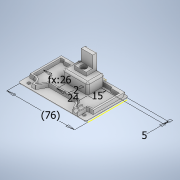
# Autodesk Inventor part: Deckel_Logo
Saved by Autodesk Inventor 2020 (Build 240168000, 168)
## iProperties
Created: 2020-09-26
Part Number: Deckel_Logo
Material: Generisch
Document SubType Name: Modeling
Designer: hpcwoess
Density: 1 g/cm^3
Appearance: Vorgabe
Author: hpcwoess
Autodesk Inventor part; units mm, degrees
ref_plane "YZ Plane" through (0, 0, 0) normal (1, 0, 0) x (0, 1, 0)
ref_plane "XY Plane" through (0, 0, 0) normal (0, 0, 1) x (1, 0, 0)
ref_plane "Arbeitsebene1" through (-34.5, -94, 30.7) normal (0, 1, 0) x (-1, 0, 0)
sketch "Skizze1" plane through (-34.5, -94, 30.7) normal (0, 1, 0) x (-1, 0, 0)
  circle A0 centre (-5, 5) radius 1.75 projected
  circle A1 centre (-67, 5) radius 1.75 projected
  arc A2 (-54.3246, 3.4866) -> (-54.0238, 3.1454) centre (-53.4437, 3.96) ccw projected
  line L0 (-54.3246, 3.4866) -> (-56.467, 7.4734) projected
  arc A3 (-56.467, 7.4734) -> (-57.3479, 8) centre (-57.3479, 7) ccw projected
  line L1 (-10, 8) -> (-14.6521, 8) projected
  arc A4 (-67, 0) -> (-65.2, 0.3352) centre (-67, 5) ccw projected
  line L2 (-67, 0) -> (-72, 0) projected
  line L3 (-72, 0) -> (-72, -34.5) projected
  line L4 (-62, -34.5) -> (-72, -34.5) projected
  line L5 (-62, -36) -> (-62, -34.5) projected
  line L6 (-62, -36) -> (-26, -36) projected
  line L7 (-26, -36) -> (-26, -34.5) projected
  line L8 (-9, -34.5) -> (-26, -34.5) projected
  line L9 (-9, -36) -> (-9, -34.5) projected
  line L10 (-9, -36) -> (-1, -36) projected
  arc A5 (-1, -36) -> (0, -35) centre (-1, -35) ccw projected
  line L11 (0, -35) -> (0, 0) projected
  line L12 (0, 0) -> (-5, 0) projected
  arc A6 (-10, 5) -> (-5, 0) centre (-5, 5) ccw projected
  line L13 (-10, 5) -> (-10, 8) projected
  arc A7 (-14.6521, 8) -> (-15.533, 7.4734) centre (-14.6521, 7) ccw projected
  line L14 (-15.533, 7.4734) -> (-20.4626, -1.7) projected
  line L15 (-24.2, -1.7) -> (-20.4626, -1.7) projected
  arc A8 (-24.2, -1.7) -> (-24.2487, -0.7) centre (-34.5, -1.7) ccw projected
  line L16 (-24.2487, -0.7) -> (-22.25, -0.7) projected
  line L17 (-22.25, 8) -> (-22.25, -0.7) projected
  line L18 (-22.25, 8) -> (-49.75, 8) projected
  line L19 (-49.75, -0.7) -> (-49.75, 8) projected
  line L20 (-49.75, -0.7) -> (-47, -0.7) projected
  line L21 (-47, -1.7) -> (-47, -0.7) projected
  line L22 (-50.4728, -1.7) -> (-47, -1.7) projected
  arc A9 (-50.4728, -1.7) -> (-54.0238, 3.1454) centre (-59.5709, -4.6437) ccw projected
  arc A10 (-74, -36) -> (-72, -38) centre (-72, -36) ccw projected
  line L23 (-74, -36) -> (-74, 8) projected
  arc A11 (-72, 10) -> (-74, 8) centre (-72, 8) ccw projected
  line L24 (-58.8, 10) -> (0, 10) projected
  arc A12 (2, 8) -> (0, 10) centre (0, 8) ccw projected
  line L25 (2, 8) -> (2, -36) projected
  arc A13 (0, -38) -> (2, -36) centre (0, -36) ccw projected
  line L26 (0, -38) -> (-72, -38) projected
  line L27 (-26.4, -35.6) -> (-61.6, -35.6)
  line L28 (-61.6, -35.6) -> (-61.6, -34.1)
  line L29 (-61.6, -34.1) -> (-71.6, -34.1)
  line L30 (-71.6, -34.1) -> (-71.6, -0.4)
  line L31 (-71.6, -0.4) -> (-67, -0.4)
  arc A14 (-67, -0.4) -> (-61.624, 4.4915) centre (-67, 5) ccw
  line L32 (-61.624, 4.4915) -> (-61.624, 7.6)
  line L33 (-61.624, 7.6) -> (-57.3479, 7.6)
  arc A15 (-56.8193, 7.284) -> (-57.3479, 7.6) centre (-57.3479, 7) ccw
  line L34 (-56.8193, 7.284) -> (-54.6769, 3.2973)
  arc A16 (-54.6769, 3.2973) -> (-54.2558, 2.8196) centre (-53.4437, 3.96) ccw
  arc A17 (-50.7686, -2.1) -> (-54.2558, 2.8196) centre (-59.5709, -4.6437) ccw
  line L35 (-50.7686, -2.1) -> (-46.6, -2.1)
  line L36 (-46.6, -2.1) -> (-46.6, -0.3)
  line L37 (-46.6, -0.3) -> (-49.35, -0.3)
  line L38 (-49.35, -0.3) -> (-49.35, 7.6)
  line L39 (-49.35, 7.6) -> (-22.65, 7.6)
  line L40 (-22.65, 7.6) -> (-22.65, -0.3)
  line L41 (-22.65, -0.3) -> (-24.6995, -0.3)
  arc A18 (-24.6081, -2.1) -> (-24.6995, -0.3) centre (-34.5, -1.7) ccw
  line L42 (-24.6081, -2.1) -> (-20.2235, -2.1)
  line L43 (-20.2235, -2.1) -> (-15.1807, 7.284)
  arc A19 (-14.6521, 7.6) -> (-15.1807, 7.284) centre (-14.6521, 7) ccw
  line L44 (-14.6521, 7.6) -> (-10.4, 7.6)
  line L45 (-10.4, 7.6) -> (-10.4, 5)
  arc A20 (-10.4, 5) -> (-5, -0.4) centre (-5, 5) ccw
  line L46 (-5, -0.4) -> (-0.4, -0.4)
  line L47 (-0.4, -0.4) -> (-0.4, -35)
  arc A21 (-1, -35.6) -> (-0.4, -35) centre (-1, -35) ccw
  line L48 (-1, -35.6) -> (-8.6, -35.6)
  line L49 (-8.6, -35.6) -> (-8.6, -34.1)
  line L50 (-8.6, -34.1) -> (-26.4, -34.1)
  line L51 (-26.4, -34.1) -> (-26.4, -35.6)
  line L52 (-59.6, -33.6) -> (-28.4, -33.6)
  line L53 (-28.4, -33.6) -> (-28.4, -32.1)
  line L54 (-28.4, -32.1) -> (-6.6, -32.1)
  line L55 (-6.6, -32.1) -> (-6.6, -33.6)
  line L56 (-6.6, -33.6) -> (-2.4, -33.6)
  line L57 (-2.4, -33.6) -> (-2.4, -2.4)
  line L58 (-2.4, -2.4) -> (-5, -2.4)
  arc A22 (-12.4, 5) -> (-5, -2.4) centre (-5, 5) ccw
  line L59 (-12.4, 5) -> (-12.4, 5.6)
  line L60 (-12.4, 5.6) -> (-13.8151, 5.6)
  line L61 (-13.8151, 5.6) -> (-19.0277, -4.1)
  line L62 (-19.0277, -4.1) -> (-26.9734, -4.1)
  arc A23 (-26.9734, -4.1) -> (-27.3691, 1.7) centre (-34.5, -1.7) ccw
  line L63 (-27.3691, 1.7) -> (-24.65, 1.7)
  line L64 (-24.65, 1.7) -> (-24.65, 5.6)
  line L65 (-24.65, 5.6) -> (-47.35, 5.6)
  line L66 (-47.35, 5.6) -> (-47.35, 1.7)
  line L67 (-47.35, 1.7) -> (-44.6, 1.7)
  line L68 (-44.6, 1.7) -> (-44.6, -4.1)
  line L69 (-44.6, -4.1) -> (-52.4291, -4.1)
  arc A24 (-52.4291, -4.1) -> (-55.416, 1.1905) centre (-59.5709, -4.6437) ccw
  arc A25 (-56.4387, 2.3505) -> (-55.416, 1.1905) centre (-53.4437, 3.96) ccw
  line L70 (-56.4387, 2.3505) -> (-58.1849, 5.6)
  line L71 (-58.1849, 5.6) -> (-59.624, 5.6)
  line L72 (-59.624, 5.6) -> (-59.624, 4.4046)
  arc A26 (-67, -2.4) -> (-59.624, 4.4046) centre (-67, 5) ccw
  line L73 (-67, -2.4) -> (-69.6, -2.4)
  line L74 (-69.6, -2.4) -> (-69.6, -32.1)
  line L75 (-69.6, -32.1) -> (-59.6, -32.1)
  line L76 (-59.6, -32.1) -> (-59.6, -33.6)
  line L77 (-65.2, 10) -> (-65.2, 0.3352) projected
  line L78 (-57.3479, 8) -> (-58.8, 8) projected
  line L79 (-58.8, 8) -> (-58.8, 10) projected
  line L80 (-72, 10) -> (-65.2, 10) projected
  line L81 (-58.8, 10) -> (-65.2, 10)
  line L82 (-58.8, 8) -> (-61.8, 8)
  line L83 (-61.8, 8) -> (-61.8, 4.5)
  point P0 (-34.5, -30.7)
  dimension "d0" = 0.4
  dimension "d1" = 2
  constraints: 106 end point, 26 point on circle, 13 centre point, 2 horizontal, 1 perpendicular, 57 other
  measures "d0" distance between parallel lines of L6 L27
  measures "d1" distance between parallel lines of L27 L52
extrude "Extrusion1" add sketch "Skizze1" against normal blind 2 contours L0 A3 L78 L79 L24 A12 L25 A13 L26 A10 L23 A11 L80 L77 A4 L2 L3 L4 L5 L6 L7 L8 L9 L10 A5 L11 L12 A6 L13 L1 A7 L14 L15 A8 L16 L17 L18 L19 L20 L21 L22 A9 A2 | A2 A9 L22 L21 L20 L19 L18 L17 L16 A8 L15 L14 A7 L1 L13 A6 L12 L11 A5 L10 L9 L8 L7 L6 L5 L4 L3 L2 A4 L77 L81 L79 L78 A3 L0 | L27 L28 L29 L30 L31 A14 L32 L33 A15 L34 A16 A17 L35 L36 L37 L38 L39 L40 L41 A18 L42 L43 A19 L44 L45 A20 L46 L47 A21 L48 L49 L50 L51 | L76 L75 L74 L73 A26 L72 L71 L70 A25 A24 L69 L68 L67 L66 L65 L64 L63 A23 L62 L61 L60 L59 A22 L58 L57 L56 L55 L54 L53 L52
sketch "Skizze4" plane through (-34.5, -94, 30.7) normal (0, 1, 0) x (-1, 0, 0)
  circle A0 centre (-5, 5) radius 1.75
  circle A1 centre (-67, 5) radius 1.75
  arc A2 (-54.3246, 3.4866) -> (-54.0238, 3.1454) centre (-53.4437, 3.96) ccw
  line L0 (-54.3246, 3.4866) -> (-56.467, 7.4734)
  arc A3 (-56.467, 7.4734) -> (-57.3479, 8) centre (-57.3479, 7) ccw
  line L1 (-57.3479, 8) -> (-62.024, 8)
  line L2 (-62.024, 8) -> (-62.024, 4.5108)
  arc A4 (-67, 0) -> (-62.024, 4.5108) centre (-67, 5) ccw
  line L3 (-67, 0) -> (-72, 0)
  line L4 (-72, 0) -> (-72, -34.5)
  line L5 (-62, -34.5) -> (-72, -34.5)
  line L6 (-62, -36) -> (-62, -34.5)
  line L7 (-62, -36) -> (-26, -36)
  line L8 (-26, -36) -> (-26, -34.5)
  line L9 (-9, -34.5) -> (-26, -34.5)
  line L10 (-9, -36) -> (-9, -34.5)
  line L11 (-9, -36) -> (-1, -36)
  arc A5 (-1, -36) -> (0, -35) centre (-1, -35) ccw
  line L12 (0, -35) -> (0, 0)
  line L13 (0, 0) -> (-5, 0)
  arc A6 (-10, 5) -> (-5, 0) centre (-5, 5) ccw
  line L14 (-10, 5) -> (-10, 8)
  line L15 (-10, 8) -> (-14.6521, 8)
  arc A7 (-14.6521, 8) -> (-15.533, 7.4734) centre (-14.6521, 7) ccw
  line L16 (-15.533, 7.4734) -> (-20.4626, -1.7)
  line L17 (-24.2, -1.7) -> (-20.4626, -1.7)
  arc A8 (-24.2, -1.7) -> (-24.2487, -0.7) centre (-34.5, -1.7) ccw
  line L18 (-24.2487, -0.7) -> (-22.25, -0.7)
  line L19 (-22.25, 8) -> (-22.25, -0.7)
  line L20 (-22.25, 8) -> (-49.75, 8)
  line L21 (-49.75, -0.7) -> (-49.75, 8)
  line L22 (-49.75, -0.7) -> (-47, -0.7)
  line L23 (-47, -1.7) -> (-47, -0.7)
  line L24 (-50.4728, -1.7) -> (-47, -1.7)
  arc A9 (-50.4728, -1.7) -> (-54.0238, 3.1454) centre (-59.5709, -4.6437) ccw
  arc A10 (-74, -36) -> (-72, -38) centre (-72, -36) ccw
  line L25 (-74, -36) -> (-74, 8)
  arc A11 (-72, 10) -> (-74, 8) centre (-72, 8) ccw
  line L26 (-72, 10) -> (0, 10)
  arc A12 (2, 8) -> (0, 10) centre (0, 8) ccw
  line L27 (2, 8) -> (2, -36)
  arc A13 (0, -38) -> (2, -36) centre (0, -36) ccw
  line L28 (0, -38) -> (-72, -38)
  line L29 (-26.4, -35.6) -> (-61.6, -35.6)
  line L30 (-61.6, -35.6) -> (-61.6, -34.1)
  line L31 (-61.6, -34.1) -> (-71.6, -34.1)
  line L32 (-71.6, -34.1) -> (-71.6, -0.4)
  line L33 (-71.6, -0.4) -> (-67, -0.4)
  arc A14 (-67, -0.4) -> (-61.624, 4.4915) centre (-67, 5) ccw
  line L34 (-61.624, 4.4915) -> (-61.624, 7.6)
  line L35 (-61.624, 7.6) -> (-57.3479, 7.6)
  arc A15 (-56.8193, 7.284) -> (-57.3479, 7.6) centre (-57.3479, 7) ccw
  line L36 (-56.8193, 7.284) -> (-54.6769, 3.2973)
  arc A16 (-54.6769, 3.2973) -> (-54.2558, 2.8196) centre (-53.4437, 3.96) ccw
  arc A17 (-50.7686, -2.1) -> (-54.2558, 2.8196) centre (-59.5709, -4.6437) ccw
  line L37 (-50.7686, -2.1) -> (-20.2235, -2.1)
  line L38 (-46.6, -0.3) -> (-49.35, -0.3)
  line L39 (-49.35, -0.3) -> (-49.35, 7.6)
  line L40 (-49.35, 7.6) -> (-22.65, 7.6)
  line L41 (-22.65, 7.6) -> (-22.65, -0.3)
  line L42 (-22.65, -0.3) -> (-24.6995, -0.3)
  line L43 (-24.6081, -2.1) -> (-20.2235, -2.1)
  line L44 (-20.2235, -2.1) -> (-15.1807, 7.284)
  arc A18 (-14.6521, 7.6) -> (-15.1807, 7.284) centre (-14.6521, 7) ccw
  line L45 (-14.6521, 7.6) -> (-10.4, 7.6)
  line L46 (-10.4, 7.6) -> (-10.4, 5)
  arc A19 (-10.4, 5) -> (-5, -0.4) centre (-5, 5) ccw
  line L47 (-5, -0.4) -> (-0.4, -0.4)
  line L48 (-0.4, -0.4) -> (-0.4, -35)
  arc A20 (-1, -35.6) -> (-0.4, -35) centre (-1, -35) ccw
  line L49 (-1, -35.6) -> (-8.6, -35.6)
  line L50 (-8.6, -35.6) -> (-8.6, -34.1)
  line L51 (-8.6, -34.1) -> (-26.4, -34.1)
  line L52 (-26.4, -34.1) -> (-26.4, -35.6)
  line L53 (-59.6, -33.6) -> (-28.4, -33.6)
  line L54 (-28.4, -33.6) -> (-28.4, -32.1)
  line L55 (-28.4, -32.1) -> (-6.6, -32.1)
  line L56 (-6.6, -32.1) -> (-6.6, -33.6)
  line L57 (-6.6, -33.6) -> (-2.4, -33.6)
  line L58 (-2.4, -33.6) -> (-2.4, -2.4)
  line L59 (-2.4, -2.4) -> (-5, -2.4)
  arc A21 (-12.4, 5) -> (-5, -2.4) centre (-5, 5) ccw
  line L60 (-12.4, 5) -> (-12.4, 5.6)
  line L61 (-12.4, 5.6) -> (-13.8151, 5.6)
  line L62 (-13.8151, 5.6) -> (-19.0277, -4.1)
  line L63 (-19.0277, -4.1) -> (-26.9734, -4.1)
  line L64 (-27.3691, 1.7) -> (-24.65, 1.7)
  line L65 (-24.65, 1.7) -> (-24.65, 5.6)
  line L66 (-24.65, 5.6) -> (-47.35, 5.6)
  line L67 (-47.35, 5.6) -> (-47.35, 1.7)
  line L68 (-47.35, 1.7) -> (-44.6, 1.7)
  line L69 (-19.0277, -4.1) -> (-52.4291, -4.1)
  arc A22 (-52.4291, -4.1) -> (-55.416, 1.1905) centre (-59.5709, -4.6437) ccw
  arc A23 (-56.4387, 2.3505) -> (-55.416, 1.1905) centre (-53.4437, 3.96) ccw
  line L70 (-56.4387, 2.3505) -> (-58.1849, 5.6)
  line L71 (-58.1849, 5.6) -> (-59.624, 5.6)
  line L72 (-59.624, 5.6) -> (-59.624, 4.4046)
  arc A24 (-67, -2.4) -> (-59.624, 4.4046) centre (-67, 5) ccw
  line L73 (-67, -2.4) -> (-69.6, -2.4)
  line L74 (-69.6, -2.4) -> (-69.6, -32.1)
  line L75 (-69.6, -32.1) -> (-59.6, -32.1)
  line L76 (-59.6, -32.1) -> (-59.6, -33.6)
  point P0 (-34.5, -30.7)
  point P1 (-34.5, -30.7)
  point P2 (-26.9734, -4.1)
  dimension "d4" = 0.4
  dimension "d5" = 2
  constraints: 154 end point, 46 point on circle, 25 centre point, 51 other
  measures "d4" distance between parallel lines of L7 L29
  measures "d5" distance between parallel lines of L29 L53
extrude "Extrusion2" add sketch "Skizze4" along normal blind 4 contours L29 L30 L31 L32 L33 A14 L34 L35 A15 L36 A16 A17 L37 L44 A18 L45 L46 A19 L47 L48 A20 L49 L50 L51 L52
sketch "Skizze5" plane through (-34.5, -96, 30.7) normal (0, -1, 0) x (1, 0, 0)
  line L0 (24, -18) -> (48, -18)
  line L1 (48, -18) -> (48, -33)
  line L2 (48, -33) -> (24, -33)
  line L3 (24, -33) -> (24, -18)
  line L4 (-2, 8) -> (-2, -36) projected
  line L5 (74, -36) -> (74, 8) projected
  line L6 (0, -38) -> (72, -38) projected
  line L7 (50, -16) -> (22, -16)
  line L8 (22, -16) -> (22, -35)
  line L9 (22, -35) -> (50, -35)
  line L10 (50, -35) -> (50, -16)
  point P0 (34.5, -30.7)
  dimension "d8" = 24
  dimension "d9" = 15
  dimension "d10" = 26
  dimension "d11" = 76
  dimension "d12" = 5
  dimension "d13" = 2
  constraints: 16 end point, 4 parallel, 2 perpendicular, 1 horizontal, 3 other
  measures "d8" distance of L0.start L0.end
  measures "d9" distance of L0.end L1.end
  measures "d10" distance between parallel lines of L4 L3
  measures "d11" distance between parallel lines of L5 L4
  measures "d12" distance between parallel lines of L2 L6
  measures "d13" distance between parallel lines of L0 L7
extrude "Extrusion3" add sketch "Skizze5" against normal blind 14 contours L0 L1 L2 L3 | L10 L9 L8 L7
extrude "Extrusion4" cut sketch "Skizze5" against normal blind 12 contours L0 L1 L2 L3
sketch "Skizze6" plane through (-34.5, -84, 30.7) normal (0, -1, 0) x (1, 0, 0)
  circle A0 centre (36, -25.5) radius 3.25
  line L0 (48, -18) -> (48, -33) projected
  line L1 (24, -18) -> (48, -18) projected
  line L2 (29.5, -21.75) -> (42.5, -21.75)
  line L3 (42.5, -21.75) -> (42.5, -29.25)
  line L4 (42.5, -29.25) -> (29.5, -29.25)
  line L5 (29.5, -29.25) -> (29.5, -21.75)
  line L6 (50, -35) -> (22, -35) projected
  line L7 (29.5, -29.25) -> (42.5, -29.25)
  line L8 (42.5, -29.25) -> (42.5, -35)
  line L9 (42.5, -35) -> (29.5, -35)
  line L10 (29.5, -35) -> (29.5, -29.25)
  point P0 (34.5, -30.7)
  dimension "d18" = 6.5
  dimension "d19" = 12
  dimension "d20" = 7.5
  dimension "d25" = 7.5
  dimension "d26" = 3.75
  dimension "d27" = 13
  dimension "d28" = 6.5
  constraints: 16 end point, 4 parallel, 2 horizontal, 2 perpendicular, 2 point on line, 1 centre point
  measures "d18" diameter of A0
  measures "d19" distance from line of A0.centre L0
  measures "d20" distance from line of L1 A0.centre
  measures "d25" distance between parallel lines of L2 L4
  measures "d26" distance from line of L4 A0.centre
  measures "d27" distance of L2.start L2.end
  measures "d28" distance from line of L3 A0.centre
sketch "Skizze7" plane through (37.1, -94, -3.4) normal (1, 0, 0) x (0, 0, -1)
  line L0 (1.5, 4) -> (0.9, 4) projected
  line L1 (3.9, 0) -> (3.9, -2) projected
  line L2 (1.5, 4) -> (3.9, 4)
  line L3 (3.9, 4) -> (3.9, 0)
  line L4 (3.9, 0) -> (1.5, 0)
  line L5 (1.5, 0) -> (1.5, 4)
  line L6 (3.9, 0) -> (2.2, 0)
  line L7 (2.2, 0) -> (2.2, 2.2)
  line L8 (2.2, 2.2) -> (3.9, 2.2)
  line L9 (3.9, 2.2) -> (3.9, 0)
  line L10 (0, 0) -> (0, 4) projected
  line L11 (1.5, 4) -> (0, 4)
  line L12 (0, 4) -> (0, 0)
  line L13 (0, 0) -> (1.5, 0)
  line L14 (1.5, 0) -> (1.5, 4)
  point P0 (-3.4, 94)
  point P1 (2.2, 0)
  point P2 (3.9, 2.2)
  point P3 (1.5, 0)
  dimension "d21" = 1.7
  dimension "d22" = 2.2
  constraints: 24 end point, 6 parallel, 3 horizontal, 3 perpendicular
  measures "d21" distance of L7.end L8.end
  measures "d22" distance of L6.end L7.end
extrude "Extrusion5" add sketch "Skizze7" against normal up to surface (71.2 mm away) contours L5 L13 L10 L11 L0 | L2 L3 L8 L7 L4 L5
sketch "Skizze8" plane through (-34.5, -96, 30.7) normal (0, -1, 0) x (1, 0, 0)
  point P0 (34.5, -30.7)
extrude "Extrusion6" add sketch "Skizze6" against normal blind 6 contours L2 L3 L4 L5
sketch "Skizze9" plane through (-34.5, -84, 30.7) normal (0, -1, 0) x (1, 0, 0)
  circle A0 centre (36, -25.5) radius 3.25
  line L0 (48, -18) -> (48, -33)
  line L1 (24, -18) -> (48, -18)
  line L2 (29.5, -21.75) -> (42.5, -21.75)
  line L3 (42.5, -21.75) -> (42.5, -29.25)
  line L4 (42.5, -29.25) -> (29.5, -29.25)
  line L5 (29.5, -29.25) -> (29.5, -21.75)
  line L6 (50, -35) -> (22, -35)
  line L7 (29.5, -29.25) -> (42.5, -29.25)
  line L8 (42.5, -29.25) -> (42.5, -35)
  line L9 (42.5, -35) -> (29.5, -35)
  line L10 (29.5, -35) -> (29.5, -29.25)
  point P0 (34.5, -30.7)
  point P1 (34.5, -30.7)
  dimension "d31" = 6.5
  dimension "d32" = 12
  dimension "d33" = 7.5
  dimension "d34" = 7.5
  dimension "d35" = 3.75
  dimension "d36" = 13
  dimension "d37" = 6.5
  constraints: 22 end point, 4 parallel, 2 horizontal, 2 perpendicular, 2 point on line, 1 centre point
  measures "d31" diameter of A0
  measures "d32" distance from line of A0.centre L0
  measures "d33" distance from line of L1 A0.centre
  measures "d34" distance between parallel lines of L2 L4
  measures "d35" distance from line of L4 A0.centre
  measures "d36" distance of L2.start L2.end
  measures "d37" distance from line of L3 A0.centre
extrude "Extrusion7" add sketch "Skizze9" against normal blind 19 contours L4 L8 L6 L10
sketch "Skizze10" plane through (-34.5, -78, 30.7) normal (0, 1, 0) x (1, 0, 0)
  line L0 (29.5, 21.75) -> (42.5, 21.75) projected
  line L1 (42.5, 21.75) -> (42.5, 29.25) projected
  line L2 (42.5, 29.25) -> (29.5, 29.25) projected
  line L3 (29.5, 29.25) -> (29.5, 21.75) projected
  circle A0 centre (36, 25.5) radius 3.25 projected
  point P0 (34.5, 30.7)
extrude "Extrusion8" cut sketch "Skizze10" against normal blind 10 contours A0
fillet "Rundung1" radius 2 20 edges at (1.5, -96, 12.7) (13.5, -96, 5.2) (1.5, -96, -2.3) (-10.5, -96, 5.2) (1.5, -82, 14.7) (15.5, -82, 5.2) (1.5, -84, -2.3) (-10.5, -84, 5.2) (1.5, -84, 12.7) (13.5, -84, 5.2) (-12.5, -82, 5.2) (15.5, -88, 14.7) (-12.5, -88, 14.7) (1.5, -65, -4.3) (8, -73.5, -4.3) (-5, -73.5, -4.3) (11.75, -82, -4.3) (-8.75, -82, -4.3) (15.5, -86, -4.3) (-12.5, -86, -4.3)
fillet "Rundung2" radius 2 7 edges at (-35.9142, -96, 40.1142) (-36.5, -96, 16.7) (-35.9142, -96, -6.7142) (1.5, -96, -7.3) (38.9142, -96, -6.7142) (39.5, -96, 16.7) (38.9142, -96, 40.1142)
sketch "Skizze11" plane through (-34.5, -84, 30.7) normal (0, -1, 0) x (1, 0, 0)
  line L0 (27.3428, -21.9377) -> (49.5374, -21.9377) construction
  line L1 (49.5374, -21.9377) -> (49.5374, -30.3697) construction
  line L2 (49.5374, -30.3697) -> (27.3428, -30.3697) construction
  line L3 (27.3428, -30.3697) -> (27.3428, -21.9377) construction
  line L4 (30.4911, -29.0852) -> (27.7796, -29.0852)
  line L5 (27.7796, -29.0852) -> (27.7796, -28.3705)
  line L6 (27.7796, -28.3705) -> (28.6702, -28.3705)
  line L7 (28.6702, -28.3705) -> (28.6702, -22.8)
  line L8 (28.6702, -22.8) -> (27.7796, -22.8)
  line L9 (27.7796, -22.8) -> (27.7796, -22.0852)
  line L10 (27.7796, -22.0852) -> (30.4911, -22.0852)
  line L11 (30.4911, -22.0852) -> (30.4911, -22.8)
  line L12 (30.4911, -22.8) -> (29.6005, -22.8)
  line L13 (29.6005, -22.8) -> (29.6005, -28.3705)
  line L14 (29.6005, -28.3705) -> (30.4911, -28.3705)
  line L15 (30.4911, -28.3705) -> (30.4911, -29.0852)
  spline S0 degree 2 poles (45.6143, -22.8851) (46.0114, -23.3502) (46.4538, -24.7116) (46.4538, -25.5852) knots 0 0 0 1 2 2 2
  spline S1 degree 2 poles (46.4538, -25.5852) (46.4538, -26.4361) (46.0227, -27.8145) (45.6143, -28.2797) knots 0 0 0 1 2 2 2
  spline S2 degree 2 poles (45.6143, -28.2797) (45.1832, -28.7675) (44.043, -29.2327) (43.3566, -29.2327) knots 0 0 0 1 2 2 2
  spline S3 degree 2 poles (43.3566, -29.2327) (42.6475, -29.2327) (41.513, -28.7505) (41.0989, -28.2797) knots 0 0 0 1 2 2 2
  spline S4 degree 2 poles (41.0989, -28.2797) (40.6961, -27.8145) (40.265, -26.4474) (40.265, -25.5852) knots 0 0 0 1 2 2 2
  spline S5 degree 2 poles (40.265, -25.5852) (40.265, -24.706) (40.7018, -23.3672) (41.1046, -22.8851) knots 0 0 0 1 2 2 2
  spline S6 degree 2 poles (41.1046, -22.8851) (41.513, -22.4199) (42.6532, -21.9377) (43.3566, -21.9377) knots 0 0 0 1 2 2 2
  spline S7 degree 2 poles (43.3566, -21.9377) (44.0714, -21.9377) (45.2172, -22.4369) (45.6143, -22.8851) knots 0 0 0 1 2 2 2
  spline S8 degree 2 poles (45.4838, -25.5852) (45.4838, -24.8932) (45.1832, -23.821) (44.9109, -23.4693) knots 0 0 0 1 2 2 2
  spline S9 degree 2 poles (44.9109, -23.4693) (44.6329, -23.1063) (43.8501, -22.7432) (43.3623, -22.7432) knots 0 0 0 1 2 2 2
  spline S10 degree 2 poles (43.3623, -22.7432) (42.8574, -22.7432) (42.0973, -23.0949) (41.808, -23.4693) knots 0 0 0 1 2 2 2
  spline S11 degree 2 poles (41.808, -23.4693) (41.53, -23.8267) (41.235, -24.9045) (41.235, -25.5852) knots 0 0 0 1 2 2 2
  spline S12 degree 2 poles (41.235, -25.5852) (41.235, -26.9637) (42.3923, -28.4272) (43.3623, -28.4272) knots 0 0 0 1 2 2 2
  spline S13 degree 2 poles (43.3623, -28.4272) (44.3323, -28.4272) (45.4838, -26.9637) (45.4838, -25.5852) knots 0 0 0 1 2 2 2
  point P0 (34.5, -30.7)
  constraints: 2 other
extrude "Extrusion9" cut sketch "Skizze11" against normal mid plane 1
chamfer "Fase1" distance 0.5 distance2 4 1 edges at (0.9961, -90, 28.6) measured on face at (0.9961, -90, 28.1)
chamfer "Fase2" distance 0.5 distance2 4 6 edges at (16.2005, -90, 28.351) (17.5959, -90, 31.3549) (19.9939, -90, 33.7342) (21.2481, -90, 35.9906) (22.54, -90, 38.215) (24.9859, -90, 38.3) measured on face at (16.6845, -90, 28.2257) measured on face at (21.6886, -90, 35.754) measured on face at (24.9859, -90, 37.8) measured on face at (18.0038, -90, 31.0658) measured on face at (22.7965, -90, 37.7858) measured on face at (20.369, -90, 33.4035)
chamfer "Fase3" distance 0.5 distance2 4 2 edges at (28.8658, -90, 31.7059) (34.8, -90, 30.3)
chamfer "Fase4" distance 0.5 distance2 4 1 edges at (27.124, -90, 35.5347) measured on face at (26.624, -90, 35.5347)
chamfer "Fase5" distance 0.5 distance2 4 3 edges at (-16.6636, -90, 33.0421) (-19.54, -90, 38.215) (-21.9739, -90, 38.3) measured on face at (-19.7965, -90, 37.7858) measured on face at (-21.9739, -90, 37.8) measured on face at (-17.104, -90, 32.8054)
chamfer "Fase6" distance 0.5 distance2 4 3 edges at (-25.6816, -90, 31.8816) (-24.1, -90, 36.75) (-31.8, -90, 30.3) measured on face at (-25.3281, -90, 31.5281) measured on face at (-23.6, -90, 36.75) measured on face at (-31.8, -90, 29.8)
sketch "Skizze12" plane through (-34.5, -94, 30.7) normal (0, 1, 0) x (1, 0, 0)
  line L0 (0, -10) -> (59, -10) projected
  line L1 (65, -10) -> (59, -10)
  line L2 (59, -10) -> (59, 0)
  line L3 (59, 0) -> (65, 0)
  line L4 (65, 0) -> (65, -10)
  circle A0 centre (67, -5) radius 1.75 projected
  point P0 (34.5, 30.7)
  point P1 (72, -10)
  dimension "d66" = 6
  dimension "d67" = 10
  dimension "d68" = 2
  constraints: 8 end point, 2 parallel, 1 horizontal, 1 perpendicular, 1 point on line
  measures "d66" distance of L2.end L3.end
  measures "d67" distance of L0.end L2.end
  measures "d68" distance from line of A0.centre L4
extrude "Extrusion10" add sketch "Skizze12" along normal blind 4 contours L1 L2 L3 L4
sketch "Skizze13" plane through (-34.5, -90, 30.7) normal (0, 1, 0) x (1, 0, 0)
  line L0 (65, -10) -> (65, 0) projected
  line L1 (59, -7.1) -> (59, -5.6) projected
  line L2 (59, -10) -> (65, -10) projected
  line L3 (62, -10) -> (62, 0)
  line L4 (65, 0) -> (63.8679, 0) projected
  line L5 (60, 0) -> (60, -10)
  line L6 (64, 0) -> (64, -10)
  line L7 (60, -4.5) -> (60.1, -4.5)
  line L8 (60.1, -4.5) -> (60.1, -5.5)
  line L9 (60.1, -5.5) -> (60, -5.5)
  line L10 (60, -5.5) -> (60, -4.5)
  line L11 (60, 0) -> (62, 0)
  line L12 (61.5447, 0) -> (59, 0) projected
  line L13 (60, -10) -> (62, -10)
  line L14 (60, 0) -> (62, 0)
  line L15 (62, 0) -> (62, 3.925)
  line L16 (62, 3.925) -> (60, 3.925)
  line L17 (60, 3.925) -> (60, 0)
  point P0 (34.5, 30.7)
  point P1 (62, 0)
  dimension "d72" = 2
  dimension "d73" = 2
  dimension "d74" = 0.1
  dimension "d75" = 1
  dimension "d76" = 4.5
  constraints: 26 end point, 4 parallel, 4 point on line, 3 perpendicular, 2 collinear, 2 horizontal, 2 vertical, 1 midpoint
  measures "d72" distance between parallel lines of L5 L3
  measures "d73" distance between parallel lines of L6 L3
  measures "d74" distance of L8.end L9.end
  measures "d75" distance of L7.end L8.end
  measures "d76" distance from line of L8.end L2
revolve "Umdrehung1" cut sketch "Skizze13" angle 360 about axis through (27.5, -90, 40.7) along (0, 0, -1) contours L5 L9 L8 L7 L11 L3 L2 | L11 L17 L16 L15
sketch "Skizze14" plane through (37.1, -94, -5.6) normal (1, 0, 0) x (0, 0, -1)
  line L0 (-2, 0) -> (-2, 2.1901)
  line L1 (-2, 2.1901) -> (-0.3, 2.1901)
  line L2 (-0.3, 2.1901) -> (-0.3, 4)
  line L3 (-0.3, 4) -> (1.7, 4)
  line L4 (1.7, 4) -> (1.7, 0)
  line L5 (1.7, 0) -> (-2.2122, 0)
  line L6 (0, 0) -> (-35.9, 0) projected
  line L7 (-44.3, 0) -> (-0.3, 0) projected
  line L8 (-35.4, 4) -> (1.7, 4) projected
  line L9 (0, 0) -> (0, 2.2) projected
  point P0 (-5.6, 94)
  point P1 (-2, 0)
  dimension "d78" = 2
  dimension "d79" = 2
  constraints: 12 end point, 3 perpendicular, 3 point on line, 1 horizontal, 1 vertical
  measures "d78" distance between parallel lines of L4 L2
  measures "d79" distance between parallel lines of L9 L0
extrude "Extrusion11" cut sketch "Skizze14" against normal through all
sketch "Skizze15" plane through (-34.5, -96, 30.7) normal (0, -1, 0) x (1, 0, 0)
  spline S0 degree 3 poles (27.6343, -10.8136) (26.4266, -10.5836) (25.5352, -9.6702) (25.0298, -8.1444) knots 0 0 0 0 1 1 1 1
  line L0 (27.6343, -10.8136) -> (26.4266, -10.5836) construction
  line L1 (26.4266, -10.5836) -> (25.5352, -9.6702) construction
  line L2 (25.5352, -9.6702) -> (25.0298, -8.1444) construction
  spline S1 degree 3 poles (25.0298, -8.1444) (24.8148, -7.4954) (24.6779, -6.7642) (24.6035, -5.8681) knots 0 0 0 0 1 1 1 1
  line L3 (25.0298, -8.1444) -> (24.8148, -7.4954) construction
  line L4 (24.8148, -7.4954) -> (24.6779, -6.7642) construction
  line L5 (24.6779, -6.7642) -> (24.6035, -5.8681) construction
  spline S2 degree 3 poles (24.6035, -5.8681) (24.5626, -5.3758) (24.5622, -1.8361) (24.603, -1.3121) knots 0 0 0 0 1 1 1 1
  line L6 (24.6035, -5.8681) -> (24.5626, -5.3758) construction
  line L7 (24.5626, -5.3758) -> (24.5622, -1.8361) construction
  line L8 (24.5622, -1.8361) -> (24.603, -1.3121) construction
  spline S3 degree 3 poles (24.603, -1.3121) (24.7756, 0.9069) (25.4417, 2.4412) (26.5559, 3.1865) knots 0 0 0 0 1 1 1 1
  line L9 (24.603, -1.3121) -> (24.7756, 0.9069) construction
  line L10 (24.7756, 0.9069) -> (25.4417, 2.4412) construction
  line L11 (25.4417, 2.4412) -> (26.5559, 3.1865) construction
  spline S4 degree 3 poles (26.5559, 3.1865) (27.0164, 3.4945) (27.4533, 3.6299) (28.0687, 3.6551) knots 0 0 0 0 1 1 1 1
  line L12 (26.5559, 3.1865) -> (27.0164, 3.4945) construction
  line L13 (27.0164, 3.4945) -> (27.4533, 3.6299) construction
  line L14 (27.4533, 3.6299) -> (28.0687, 3.6551) construction
  spline S5 degree 3 poles (28.0687, 3.6551) (28.9563, 3.6916) (29.6519, 3.4344) (30.2654, 2.843) knots 0 0 0 0 1 1 1 1
  line L15 (28.0687, 3.6551) -> (28.9563, 3.6916) construction
  line L16 (28.9563, 3.6916) -> (29.6519, 3.4344) construction
  line L17 (29.6519, 3.4344) -> (30.2654, 2.843) construction
  spline S6 degree 3 poles (30.2654, 2.843) (31.0709, 2.0665) (31.5427, 0.8871) (31.7624, -0.8987) knots 0 0 0 0 1 1 1 1
  line L18 (30.2654, 2.843) -> (31.0709, 2.0665) construction
  line L19 (31.0709, 2.0665) -> (31.5427, 0.8871) construction
  line L20 (31.5427, 0.8871) -> (31.7624, -0.8987) construction
  spline S7 degree 3 poles (31.7624, -0.8987) (31.826, -1.415) (31.8567, -4.9957) (31.804, -5.7438) knots 0 0 0 0 1 1 1 1
  line L21 (31.7624, -0.8987) -> (31.826, -1.415) construction
  line L22 (31.826, -1.415) -> (31.8567, -4.9957) construction
  line L23 (31.8567, -4.9957) -> (31.804, -5.7438) construction
  spline S8 degree 3 poles (31.804, -5.7438) (31.6515, -7.9101) (31.0546, -9.4228) (30.0306, -10.2379) knots 0 0 0 0 1 1 1 1
  line L24 (31.804, -5.7438) -> (31.6515, -7.9101) construction
  line L25 (31.6515, -7.9101) -> (31.0546, -9.4228) construction
  line L26 (31.0546, -9.4228) -> (30.0306, -10.2379) construction
  spline S9 degree 3 poles (30.0306, -10.2379) (29.767, -10.4478) (29.2918, -10.6867) (28.9725, -10.7699) knots 0 0 0 0 1 1 1 1
  line L27 (30.0306, -10.2379) -> (29.767, -10.4478) construction
  line L28 (29.767, -10.4478) -> (29.2918, -10.6867) construction
  line L29 (29.2918, -10.6867) -> (28.9725, -10.7699) construction
  spline S10 degree 3 poles (28.9725, -10.7699) (28.6662, -10.8498) (27.9477, -10.8732) (27.6343, -10.8136) knots 0 0 0 0 1 1 1 1
  line L30 (28.9725, -10.7699) -> (28.6662, -10.8498) construction
  line L31 (28.6662, -10.8498) -> (27.9477, -10.8732) construction
  line L32 (27.9477, -10.8732) -> (27.6343, -10.8136) construction
  spline S11 degree 3 poles (28.652, -7.9213) (29.17, -7.6663) (29.4654, -6.9581) (29.5787, -5.6993) knots 0 0 0 0 1 1 1 1
  line L33 (28.652, -7.9213) -> (29.17, -7.6663) construction
  line L34 (29.17, -7.6663) -> (29.4654, -6.9581) construction
  line L35 (29.4654, -6.9581) -> (29.5787, -5.6993) construction
  spline S12 degree 3 poles (29.5787, -5.6993) (29.6187, -5.2557) (29.6187, -1.935) (29.5787, -1.4914) knots 0 0 0 0 1 1 1 1
  line L36 (29.5787, -5.6993) -> (29.6187, -5.2557) construction
  line L37 (29.6187, -5.2557) -> (29.6187, -1.935) construction
  line L38 (29.6187, -1.935) -> (29.5787, -1.4914) construction
  spline S13 degree 3 poles (29.5787, -1.4914) (29.4642, -0.2189) (29.1712, 0.475) (28.6378, 0.7376) knots 0 0 0 0 1 1 1 1
  line L39 (29.5787, -1.4914) -> (29.4642, -0.2189) construction
  line L40 (29.4642, -0.2189) -> (29.1712, 0.475) construction
  line L41 (29.1712, 0.475) -> (28.6378, 0.7376) construction
  spline S14 degree 3 poles (28.6378, 0.7376) (28.4636, 0.8234) (28.4123, 0.8347) (28.2027, 0.834) knots 0 0 0 0 1 1 1 1
  line L42 (28.6378, 0.7376) -> (28.4636, 0.8234) construction
  line L43 (28.4636, 0.8234) -> (28.4123, 0.8347) construction
  line L44 (28.4123, 0.8347) -> (28.2027, 0.834) construction
  spline S15 degree 3 poles (28.2027, 0.834) (27.4794, 0.8315) (27.0606, 0.2365) (26.8619, -1.0707) knots 0 0 0 0 1 1 1 1
  line L45 (28.2027, 0.834) -> (27.4794, 0.8315) construction
  line L46 (27.4794, 0.8315) -> (27.0606, 0.2365) construction
  line L47 (27.0606, 0.2365) -> (26.8619, -1.0707) construction
  spline S16 degree 3 poles (26.8619, -1.0707) (26.8151, -1.379) (26.8093, -1.6581) (26.8093, -3.5954) knots 0 0 0 0 1 1 1 1
  line L48 (26.8619, -1.0707) -> (26.8151, -1.379) construction
  line L49 (26.8151, -1.379) -> (26.8093, -1.6581) construction
  line L50 (26.8093, -1.6581) -> (26.8093, -3.5954) construction
  spline S17 degree 3 poles (26.8093, -3.5954) (26.8093, -5.5391) (26.815, -5.811) (26.8624, -6.1231) knots 0 0 0 0 1 1 1 1
  line L51 (26.8093, -3.5954) -> (26.8093, -5.5391) construction
  line L52 (26.8093, -5.5391) -> (26.815, -5.811) construction
  line L53 (26.815, -5.811) -> (26.8624, -6.1231) construction
  spline S18 degree 3 poles (26.8624, -6.1231) (27.0654, -7.4604) (27.5268, -8.0814) (28.2761, -8.0258) knots 0 0 0 0 1 1 1 1
  line L54 (26.8624, -6.1231) -> (27.0654, -7.4604) construction
  line L55 (27.0654, -7.4604) -> (27.5268, -8.0814) construction
  line L56 (27.5268, -8.0814) -> (28.2761, -8.0258) construction
  spline S19 degree 3 poles (28.2761, -8.0258) (28.4091, -8.016) (28.5255, -7.9836) (28.652, -7.9213) knots 0 0 0 0 1 1 1 1
  line L57 (28.2761, -8.0258) -> (28.4091, -8.016) construction
  line L58 (28.4091, -8.016) -> (28.5255, -7.9836) construction
  line L59 (28.5255, -7.9836) -> (28.652, -7.9213) construction
  spline S20 degree 3 poles (43.9399, -10.8094) (42.7104, -10.642) (41.7982, -9.9726) (41.1212, -8.741) knots 0 0 0 0 1 1 1 1
  line L60 (43.9399, -10.8094) -> (42.7104, -10.642) construction
  line L61 (42.7104, -10.642) -> (41.7982, -9.9726) construction
  line L62 (41.7982, -9.9726) -> (41.1212, -8.741) construction
  spline S21 degree 3 poles (41.7789, -7.7257) (42.2, -7.2754) (42.5726, -6.8729) (42.6068, -6.8312) knots 0 0 0 0 1 1 1 1
  line L63 (41.7789, -7.7257) -> (42.2, -7.2754) construction
  line L64 (42.2, -7.2754) -> (42.5726, -6.8729) construction
  line L65 (42.5726, -6.8729) -> (42.6068, -6.8312) construction
  line L66 (41.1212, -8.741) -> (41.0132, -8.5444)
  line L67 (41.0132, -8.5444) -> (41.7789, -7.7257)
  spline S22 degree 3 poles (42.7918, -6.9623) (43.1927, -7.6371) (43.7007, -7.979) (44.3757, -8.0284) knots 0 0 0 0 1 1 1 1
  line L68 (42.7918, -6.9623) -> (43.1927, -7.6371) construction
  line L69 (43.1927, -7.6371) -> (43.7007, -7.979) construction
  line L70 (43.7007, -7.979) -> (44.3757, -8.0284) construction
  spline S23 degree 3 poles (44.3757, -8.0284) (44.8325, -8.0617) (45.1907, -7.9391) (45.4299, -7.6674) knots 0 0 0 0 1 1 1 1
  line L71 (44.3757, -8.0284) -> (44.8325, -8.0617) construction
  line L72 (44.8325, -8.0617) -> (45.1907, -7.9391) construction
  line L73 (45.1907, -7.9391) -> (45.4299, -7.6674) construction
  spline S24 degree 3 poles (45.4299, -7.6674) (45.6121, -7.4604) (45.6786, -7.2585) (45.6938, -6.8658) knots 0 0 0 0 1 1 1 1
  line L74 (45.4299, -7.6674) -> (45.6121, -7.4604) construction
  line L75 (45.6121, -7.4604) -> (45.6786, -7.2585) construction
  line L76 (45.6786, -7.2585) -> (45.6938, -6.8658) construction
  spline S25 degree 3 poles (45.6938, -6.8658) (45.7143, -6.3413) (45.601, -6.0436) (45.2576, -5.7198) knots 0 0 0 0 1 1 1 1
  line L77 (45.6938, -6.8658) -> (45.7143, -6.3413) construction
  line L78 (45.7143, -6.3413) -> (45.601, -6.0436) construction
  line L79 (45.601, -6.0436) -> (45.2576, -5.7198) construction
  spline S26 degree 3 poles (45.2576, -5.7198) (44.9946, -5.4718) (44.7228, -5.2979) (44.056, -4.9511) knots 0 0 0 0 1 1 1 1
  line L80 (45.2576, -5.7198) -> (44.9946, -5.4718) construction
  line L81 (44.9946, -5.4718) -> (44.7228, -5.2979) construction
  line L82 (44.7228, -5.2979) -> (44.056, -4.9511) construction
  spline S27 degree 3 poles (44.056, -4.9511) (43.4262, -4.6236) (43.0347, -4.3719) (42.7128, -4.0876) knots 0 0 0 0 1 1 1 1
  line L83 (44.056, -4.9511) -> (43.4262, -4.6236) construction
  line L84 (43.4262, -4.6236) -> (43.0347, -4.3719) construction
  line L85 (43.0347, -4.3719) -> (42.7128, -4.0876) construction
  spline S28 degree 3 poles (42.7128, -4.0876) (41.8233, -3.3021) (41.3995, -2.3251) (41.3166, -0.8691) knots 0 0 0 0 1 1 1 1
  line L86 (42.7128, -4.0876) -> (41.8233, -3.3021) construction
  line L87 (41.8233, -3.3021) -> (41.3995, -2.3251) construction
  line L88 (41.3995, -2.3251) -> (41.3166, -0.8691) construction
  spline S29 degree 3 poles (41.3166, -0.8691) (41.2249, 0.7433) (41.5758, 2.0088) (42.3337, 2.7988) knots 0 0 0 0 1 1 1 1
  line L89 (41.3166, -0.8691) -> (41.2249, 0.7433) construction
  line L90 (41.2249, 0.7433) -> (41.5758, 2.0088) construction
  line L91 (41.5758, 2.0088) -> (42.3337, 2.7988) construction
  spline S30 degree 3 poles (42.3337, 2.7988) (42.8989, 3.3879) (43.6079, 3.6654) (44.5448, 3.6641) knots 0 0 0 0 1 1 1 1
  line L92 (42.3337, 2.7988) -> (42.8989, 3.3879) construction
  line L93 (42.8989, 3.3879) -> (43.6079, 3.6654) construction
  line L94 (43.6079, 3.6654) -> (44.5448, 3.6641) construction
  spline S31 degree 3 poles (44.5448, 3.6641) (45.176, 3.6632) (45.6072, 3.567) (46.1302, 3.3104) knots 0 0 0 0 1 1 1 1
  line L95 (44.5448, 3.6641) -> (45.176, 3.6632) construction
  line L96 (45.176, 3.6632) -> (45.6072, 3.567) construction
  line L97 (45.6072, 3.567) -> (46.1302, 3.3104) construction
  spline S32 degree 3 poles (46.1302, 3.3104) (46.6624, 3.0493) (47.0096, 2.7506) (47.3971, 2.2208) knots 0 0 0 0 1 1 1 1
  line L98 (46.1302, 3.3104) -> (46.6624, 3.0493) construction
  line L99 (46.6624, 3.0493) -> (47.0096, 2.7506) construction
  line L100 (47.0096, 2.7506) -> (47.3971, 2.2208) construction
  spline S33 degree 3 poles (47.3971, 2.2208) (47.5403, 2.025) (47.8741, 1.3978) (47.8583, 1.3543) knots 0 0 0 0 1 1 1 1
  line L101 (47.3971, 2.2208) -> (47.5403, 2.025) construction
  line L102 (47.5403, 2.025) -> (47.8741, 1.3978) construction
  line L103 (47.8741, 1.3978) -> (47.8583, 1.3543) construction
  spline S34 degree 3 poles (47.8583, 1.3543) (47.8451, 1.318) (46.254, -0.4247) (46.2348, -0.4239) knots 0 0 0 0 1 1 1 1
  line L104 (47.8583, 1.3543) -> (47.8451, 1.318) construction
  line L105 (47.8451, 1.318) -> (46.254, -0.4247) construction
  line L106 (46.254, -0.4247) -> (46.2348, -0.4239) construction
  spline S35 degree 3 poles (46.2348, -0.4239) (46.2261, -0.4235) (46.1543, -0.2891) (46.075, -0.1251) knots 0 0 0 0 1 1 1 1
  line L107 (46.2348, -0.4239) -> (46.2261, -0.4235) construction
  line L108 (46.2261, -0.4235) -> (46.1543, -0.2891) construction
  line L109 (46.1543, -0.2891) -> (46.075, -0.1251) construction
  spline S36 degree 3 poles (46.075, -0.1251) (45.8453, 0.3501) (45.5437, 0.6366) (45.141, 0.7619) knots 0 0 0 0 1 1 1 1
  line L110 (46.075, -0.1251) -> (45.8453, 0.3501) construction
  line L111 (45.8453, 0.3501) -> (45.5437, 0.6366) construction
  line L112 (45.5437, 0.6366) -> (45.141, 0.7619) construction
  spline S37 degree 3 poles (45.141, 0.7619) (44.5747, 0.9382) (44.0145, 0.8201) (43.7611, 0.4711) knots 0 0 0 0 1 1 1 1
  line L113 (45.141, 0.7619) -> (44.5747, 0.9382) construction
  line L114 (44.5747, 0.9382) -> (44.0145, 0.8201) construction
  line L115 (44.0145, 0.8201) -> (43.7611, 0.4711) construction
  spline S38 degree 3 poles (43.7611, 0.4711) (43.5212, 0.1408) (43.4539, -0.4846) (43.6107, -0.9271) knots 0 0 0 0 1 1 1 1
  line L116 (43.7611, 0.4711) -> (43.5212, 0.1408) construction
  line L117 (43.5212, 0.1408) -> (43.4539, -0.4846) construction
  line L118 (43.4539, -0.4846) -> (43.6107, -0.9271) construction
  spline S39 degree 3 poles (43.6107, -0.9271) (43.7752, -1.3913) (44.2641, -1.7974) (45.1134, -2.1752) knots 0 0 0 0 1 1 1 1
  line L119 (43.6107, -0.9271) -> (43.7752, -1.3913) construction
  line L120 (43.7752, -1.3913) -> (44.2641, -1.7974) construction
  line L121 (44.2641, -1.7974) -> (45.1134, -2.1752) construction
  spline S40 degree 3 poles (45.1134, -2.1752) (46.7138, -2.8871) (47.4692, -3.6922) (47.7776, -5.0147) knots 0 0 0 0 1 1 1 1
  line L122 (45.1134, -2.1752) -> (46.7138, -2.8871) construction
  line L123 (46.7138, -2.8871) -> (47.4692, -3.6922) construction
  line L124 (47.4692, -3.6922) -> (47.7776, -5.0147) construction
  spline S41 degree 3 poles (47.7776, -5.0147) (47.9701, -5.8403) (47.9751, -7.2371) (47.7888, -8.1368) knots 0 0 0 0 1 1 1 1
  line L125 (47.7776, -5.0147) -> (47.9701, -5.8403) construction
  line L126 (47.9701, -5.8403) -> (47.9751, -7.2371) construction
  line L127 (47.9751, -7.2371) -> (47.7888, -8.1368) construction
  spline S42 degree 3 poles (47.7888, -8.1368) (47.528, -9.3959) (46.8184, -10.3156) (45.8303, -10.6751) knots 0 0 0 0 1 1 1 1
  line L128 (47.7888, -8.1368) -> (47.528, -9.3959) construction
  line L129 (47.528, -9.3959) -> (46.8184, -10.3156) construction
  line L130 (46.8184, -10.3156) -> (45.8303, -10.6751) construction
  spline S43 degree 3 poles (45.8303, -10.6751) (45.3485, -10.8504) (44.6206, -10.9021) (43.9399, -10.8094) knots 0 0 0 0 1 1 1 1
  line L131 (45.8303, -10.6751) -> (45.3485, -10.8504) construction
  line L132 (45.3485, -10.8504) -> (44.6206, -10.9021) construction
  line L133 (44.6206, -10.9021) -> (43.9399, -10.8094) construction
  line L134 (42.6068, -6.8312) -> (42.669, -6.7555)
  line L135 (42.669, -6.7555) -> (42.7918, -6.9623)
  spline S44 degree 3 poles (35.0547, 3.4573) (36.1804, 3.4572) (36.9549, 3.445) (37.1217, 3.4246) knots 0 0 0 0 1 1 1 1
  line L136 (35.0547, 3.4573) -> (36.1804, 3.4572) construction
  line L137 (36.1804, 3.4572) -> (36.9549, 3.445) construction
  line L138 (36.9549, 3.445) -> (37.1217, 3.4246) construction
  spline S45 degree 3 poles (37.1217, 3.4246) (38.5186, 3.2541) (39.426, 2.4723) (39.7558, 1.1551) knots 0 0 0 0 1 1 1 1
  line L139 (37.1217, 3.4246) -> (38.5186, 3.2541) construction
  line L140 (38.5186, 3.2541) -> (39.426, 2.4723) construction
  line L141 (39.426, 2.4723) -> (39.7558, 1.1551) construction
  spline S46 degree 3 poles (39.7558, 1.1551) (39.8814, 0.6533) (39.905, 0.4262) (39.9044, -0.2764) knots 0 0 0 0 1 1 1 1
  line L142 (39.7558, 1.1551) -> (39.8814, 0.6533) construction
  line L143 (39.8814, 0.6533) -> (39.905, 0.4262) construction
  line L144 (39.905, 0.4262) -> (39.9044, -0.2764) construction
  spline S47 degree 3 poles (39.9044, -0.2764) (39.9038, -0.9979) (39.8703, -1.2839) (39.7293, -1.7703) knots 0 0 0 0 1 1 1 1
  line L145 (39.9044, -0.2764) -> (39.9038, -0.9979) construction
  line L146 (39.9038, -0.9979) -> (39.8703, -1.2839) construction
  line L147 (39.8703, -1.2839) -> (39.7293, -1.7703) construction
  spline S48 degree 3 poles (39.7293, -1.7703) (39.5921, -2.2437) (39.3705, -2.6512) (39.0372, -3.0433) knots 0 0 0 0 1 1 1 1
  line L148 (39.7293, -1.7703) -> (39.5921, -2.2437) construction
  line L149 (39.5921, -2.2437) -> (39.3705, -2.6512) construction
  line L150 (39.3705, -2.6512) -> (39.0372, -3.0433) construction
  line L151 (33.2545, -3.5954) -> (33.2545, 3.4574)
  line L152 (33.2545, 3.4574) -> (35.0547, 3.4573)
  spline S49 degree 3 poles (39.1628, -3.4878) (39.5484, -3.8692) (39.7879, -4.2564) (39.9626, -4.7807) knots 0 0 0 0 1 1 1 1
  line L153 (39.1628, -3.4878) -> (39.5484, -3.8692) construction
  line L154 (39.5484, -3.8692) -> (39.7879, -4.2564) construction
  line L155 (39.7879, -4.2564) -> (39.9626, -4.7807) construction
  spline S50 degree 3 poles (39.9626, -4.7807) (40.2826, -5.7406) (40.2957, -7.228) (39.9937, -8.2922) knots 0 0 0 0 1 1 1 1
  line L156 (39.9626, -4.7807) -> (40.2826, -5.7406) construction
  line L157 (40.2826, -5.7406) -> (40.2957, -7.228) construction
  line L158 (40.2957, -7.228) -> (39.9937, -8.2922) construction
  spline S51 degree 3 poles (39.9937, -8.2922) (39.9046, -8.6063) (39.6836, -9.0845) (39.5081, -9.3429) knots 0 0 0 0 1 1 1 1
  line L159 (39.9937, -8.2922) -> (39.9046, -8.6063) construction
  line L160 (39.9046, -8.6063) -> (39.6836, -9.0845) construction
  line L161 (39.6836, -9.0845) -> (39.5081, -9.3429) construction
  spline S52 degree 3 poles (39.5081, -9.3429) (39.1142, -9.9229) (38.4982, -10.3518) (37.8042, -10.5293) knots 0 0 0 0 1 1 1 1
  line L162 (39.5081, -9.3429) -> (39.1142, -9.9229) construction
  line L163 (39.1142, -9.9229) -> (38.4982, -10.3518) construction
  line L164 (38.4982, -10.3518) -> (37.8042, -10.5293) construction
  spline S53 degree 3 poles (37.8042, -10.5293) (37.3766, -10.6387) (37.1694, -10.6481) (35.1934, -10.6481) knots 0 0 0 0 1 1 1 1
  line L165 (37.8042, -10.5293) -> (37.3766, -10.6387) construction
  line L166 (37.3766, -10.6387) -> (37.1694, -10.6481) construction
  line L167 (37.1694, -10.6481) -> (35.1934, -10.6481) construction
  line L168 (39.0372, -3.0433) -> (38.8892, -3.2172)
  line L169 (38.8892, -3.2172) -> (39.1628, -3.4878)
  spline S54 degree 3 poles (36.9358, -7.7896) (37.6172, -7.6452) (37.944, -7.2163) (37.9864, -6.4105) knots 0 0 0 0 1 1 1 1
  line L170 (36.9358, -7.7896) -> (37.6172, -7.6452) construction
  line L171 (37.6172, -7.6452) -> (37.944, -7.2163) construction
  line L172 (37.944, -7.2163) -> (37.9864, -6.4105) construction
  spline S55 degree 3 poles (37.9864, -6.4105) (38.0171, -5.8269) (37.8706, -5.3235) (37.602, -5.0894) knots 0 0 0 0 1 1 1 1
  line L173 (37.9864, -6.4105) -> (38.0171, -5.8269) construction
  line L174 (38.0171, -5.8269) -> (37.8706, -5.3235) construction
  line L175 (37.8706, -5.3235) -> (37.602, -5.0894) construction
  spline S56 degree 3 poles (37.602, -5.0894) (37.2975, -4.8241) (36.9724, -4.7511) (36.0967, -4.7511) knots 0 0 0 0 1 1 1 1
  line L176 (37.602, -5.0894) -> (37.2975, -4.8241) construction
  line L177 (37.2975, -4.8241) -> (36.9724, -4.7511) construction
  line L178 (36.9724, -4.7511) -> (36.0967, -4.7511) construction
  line L179 (35.1934, -10.6481) -> (33.2545, -10.6481)
  line L180 (33.2545, -10.6481) -> (33.2545, -3.5954)
  spline S57 degree 3 poles (36.1067, -7.8324) (36.5371, -7.8321) (36.7996, -7.8185) (36.9358, -7.7897) knots 0 0 0 0 1 1 1 1
  line L181 (36.1067, -7.8324) -> (36.5371, -7.8321) construction
  line L182 (36.5371, -7.8321) -> (36.7996, -7.8185) construction
  line L183 (36.7996, -7.8185) -> (36.9358, -7.7897) construction
  line L184 (36.0967, -4.7511) -> (35.477, -4.7511)
  line L185 (35.477, -4.7511) -> (35.477, -6.292)
  line L186 (35.477, -6.292) -> (35.477, -7.8329)
  line L187 (35.477, -7.8329) -> (36.1067, -7.8324)
  spline S58 degree 3 poles (37.0239, -1.822) (37.5031, -1.6318) (37.7347, -1.1718) (37.6897, -0.5001) knots 0 0 0 0 1 1 1 1
  line L188 (37.0239, -1.822) -> (37.5031, -1.6318) construction
  line L189 (37.5031, -1.6318) -> (37.7347, -1.1718) construction
  line L190 (37.7347, -1.1718) -> (37.6897, -0.5001) construction
  spline S59 degree 3 poles (37.6897, -0.5001) (37.6455, 0.1609) (37.3712, 0.487) (36.7517, 0.615) knots 0 0 0 0 1 1 1 1
  line L191 (37.6897, -0.5001) -> (37.6455, 0.1609) construction
  line L192 (37.6455, 0.1609) -> (37.3712, 0.487) construction
  line L193 (37.3712, 0.487) -> (36.7517, 0.615) construction
  spline S60 degree 3 poles (36.7517, 0.615) (36.6781, 0.6302) (36.3612, 0.6512) (36.0475, 0.6617) knots 0 0 0 0 1 1 1 1
  line L194 (36.7517, 0.615) -> (36.6781, 0.6302) construction
  line L195 (36.6781, 0.6302) -> (36.3612, 0.6512) construction
  line L196 (36.3612, 0.6512) -> (36.0475, 0.6617) construction
  spline S61 degree 3 poles (36.166, -1.9001) (36.7975, -1.89) (36.8691, -1.8835) (37.0239, -1.822) knots 0 0 0 0 1 1 1 1
  line L197 (36.166, -1.9001) -> (36.7975, -1.89) construction
  line L198 (36.7975, -1.89) -> (36.8691, -1.8835) construction
  line L199 (36.8691, -1.8835) -> (37.0239, -1.822) construction
  line L200 (36.0475, 0.6617) -> (35.477, 0.6808)
  line L201 (35.477, 0.6808) -> (35.477, -0.6151)
  line L202 (35.477, -0.6151) -> (35.477, -1.911)
  line L203 (35.477, -1.911) -> (36.166, -1.9001)
  line L204 (13.7854, -3.3435) -> (13.7854, 1.4127)
  line L205 (13.7854, 1.4127) -> (15.193, 1.4127)
  line L206 (15.193, 1.4127) -> (16.6006, 1.4127)
  line L207 (16.6006, 1.4127) -> (16.6006, -0.2616)
  line L208 (16.6006, -0.2616) -> (16.6006, -1.9359)
  line L209 (16.6006, -1.9359) -> (19.475, -1.9359)
  line L210 (19.475, -1.9359) -> (22.3495, -1.9359)
  line L211 (22.3495, -1.9359) -> (22.3495, -3.3435)
  line L212 (22.3495, -3.3435) -> (22.3495, -4.7511)
  line L213 (22.3495, -4.7511) -> (19.475, -4.7511)
  line L214 (19.475, -4.7511) -> (16.6006, -4.7511)
  line L215 (16.6006, -4.7511) -> (16.6006, -6.4253)
  line L216 (16.6006, -6.4253) -> (16.6006, -8.0996)
  line L217 (16.6006, -8.0996) -> (15.193, -8.0996)
  line L218 (15.193, -8.0996) -> (13.7854, -8.0996)
  line L219 (13.7854, -8.0996) -> (13.7854, -3.3435)
  line L220 (55.5091, -6.4253) -> (55.5091, -4.7511)
  line L221 (55.5091, -4.7511) -> (52.6347, -4.7511)
  line L222 (52.6347, -4.7511) -> (49.7603, -4.7511)
  line L223 (49.7603, -4.7511) -> (49.7603, -3.3435)
  line L224 (49.7603, -3.3435) -> (49.7603, -1.9359)
  line L225 (49.7603, -1.9359) -> (52.6347, -1.9359)
  line L226 (52.6347, -1.9359) -> (55.5091, -1.9359)
  line L227 (55.5091, -1.9359) -> (55.5091, -0.2616)
  line L228 (55.5091, -0.2616) -> (55.5091, 1.4127)
  line L229 (55.5091, 1.4127) -> (56.9167, 1.4127)
  line L230 (56.9167, 1.4127) -> (58.3243, 1.4127)
  line L231 (58.3243, 1.4127) -> (58.3243, -3.3435)
  line L232 (58.3243, -3.3435) -> (58.3243, -8.0996)
  line L233 (58.3243, -8.0996) -> (56.9167, -8.0996)
  line L234 (56.9167, -8.0996) -> (55.5091, -8.0996)
  line L235 (55.5091, -8.0996) -> (55.5091, -6.4253)
  point P0 (34.5, -30.7)
  point P1 (13.7854, 1.4127)
  point P2 (13.7854, -3.3435)
  point P3 (16.6006, -6.4253)
  point P4 (16.6006, -4.7511)
  point P5 (19.475, -4.7511)
  point P6 (22.3495, -4.7511)
  point P7 (16.6006, -0.2616)
  point P8 (15.193, 1.4127)
  point P9 (31.804, -5.7438)
  point P10 (31.7624, -0.8987)
  point P11 (30.2654, 2.843)
  point P12 (28.0687, 3.6551)
  point P13 (26.5559, 3.1865)
  point P14 (24.6035, -5.8681)
  point P15 (26.8619, -1.0707)
  point P16 (28.6378, 0.7376)
  point P17 (29.5787, -1.4914)
  point P18 (29.5787, -5.6993)
  point P19 (28.652, -7.9213)
  point P20 (26.8624, -6.1231)
  point P21 (37.1217, 3.4246)
  point P22 (35.0547, 3.4573)
  point P23 (33.2545, 3.4574)
  point P24 (35.1934, -10.6481)
  point P25 (39.5081, -9.3429)
  point P26 (39.9937, -8.2922)
  point P27 (39.9626, -4.7807)
  point P28 (39.0372, -3.0433)
  point P29 (35.477, 0.6808)
  point P30 (36.7517, 0.615)
  point P31 (37.6897, -0.5001)
  point P32 (37.602, -5.0894)
  point P33 (37.9864, -6.4105)
  point P34 (36.9358, -7.7896)
  point P35 (36.1067, -7.8324)
  point P36 (35.477, -7.8329)
  point P37 (35.477, -6.292)
  point P38 (35.477, -4.7511)
  point P39 (36.0967, -4.7511)
  point P40 (46.075, -0.1251)
  point P41 (47.8583, 1.3543)
  point P42 (44.5448, 3.6641)
  point P43 (42.3337, 2.7988)
  point P44 (44.056, -4.9511)
  point P45 (45.2576, -5.7198)
  point P46 (45.6938, -6.8658)
  point P47 (45.4299, -7.6674)
  point P48 (44.3757, -8.0284)
  point P49 (42.7918, -6.9623)
  point P50 (42.669, -6.7555)
  point P51 (42.6068, -6.8312)
  point P52 (41.7789, -7.7257)
  point P53 (41.0132, -8.5444)
  point P54 (41.1212, -8.741)
  point P55 (47.7888, -8.1368)
  point P56 (47.7776, -5.0147)
  point P57 (45.1134, -2.1752)
  point P58 (45.141, 0.7619)
  point P59 (55.5091, -0.2616)
  point P60 (49.7603, -4.7511)
  point P61 (52.6347, -4.7511)
  point P62 (55.5091, -4.7511)
  point P63 (55.5091, -6.4253)
  constraints: 100 end point, 186 other
extrude "Extrusion12" cut sketch "Skizze15" against normal blind 0.6
equation "\"d10\" = -0.5 * d8 + 0.5 * d11"
equation "\"d19\" = 0.5 * d8"
equation "\"d20\" = 0.5 * d9"
equation "\"d26\" = 0.5 * d25"
equation "\"d28\" = 0.5 * d27"
equation "\"d32\" = 0.5 * d38"
equation "\"d33\" = 0.5 * d39"
equation "\"d35\" = 0.5 * d34"
equation "\"d37\" = 0.5 * d36"
equation "\"d73\" = d72"
equation "\"d79\" = d78"
equation "\"d38\" = 24"
equation "\"d39\" = 15"
